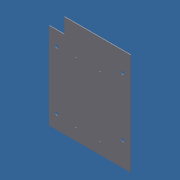
# Autodesk Inventor part: front right plate
Saved by Autodesk Inventor 2012 (Build 160160000, 160)
## iProperties
Created: 2012-03-30
Part Number: front right plate
Material: Aluminum-6061
Document SubType Name: Modeling
Designer: Edward
Density: 2.71 g/cm^3
Mass: 236.544 g
Surface Area: 1117.59 cm^2
Volume: 87.2854 cm^3
Author: Edward
Autodesk Inventor part; units mm, degrees
ref_plane "YZ Plane" through (0, 0, 0) normal (1, 0, 0) x (0, 1, 0)
ref_plane "XZ Plane" through (0, 0, 0) normal (0, 1, 0) x (-1, 0, 0)
ref_plane "XY Plane" through (0, 0, 0) normal (0, 0, 1) x (1, 0, 0)
sketch "Sketch1" plane through (0, 0, 0) normal (0, 0, 1) x (1, 0, 0)
  line L0 (0, 0) -> (213.35, 0)
  line L1 (213.35, 0) -> (213.35, 266.7)
  line L2 (213.35, 266.7) -> (0, 266.7)
  line L3 (0, 266.7) -> (0, 0)
  line L4 (0, 0) -> (41.275, 0)
  line L5 (0, 41.275) -> (0, 0)
  line L6 (0, 266.7) -> (40, 266.7)
  line L7 (40, 266.7) -> (40, 226.7)
  line L8 (40, 226.7) -> (0, 226.7)
  line L9 (0, 226.7) -> (0, 266.7)
  dimension "d0" = 266.7
  dimension "d1" = 213.35
  dimension "d4" = 40
  constraints: 20 end point, 4 parallel, 3 horizontal, 3 perpendicular
  measures "d0" distance of L2.end L0.start
  measures "d1" distance of L0.start L0.end
  measures "d4" distance of L6.end L7.end
extrude "Extrusion1" add sketch "Sketch1" along normal blind 1.5875 contours L3 L8 L7 L2 L1 L0
sketch "Sketch2" plane through (0, 0, 1.5875) normal (0, 0, 1) x (1, 0, 0)
  line L0 (213.35, 0) -> (0, 0)
  line L1 (213.35, 266.7) -> (213.35, 0)
  line L2 (40, 266.7) -> (213.35, 266.7)
  line L3 (20, 189.55) -> (20, 37.15)
  line L4 (40, 266.7) -> (40, 226.7) projected
  line L5 (40, 266.7) -> (213.35, 266.7) projected
  line L6 (0, 0) -> (0, 226.7)
  line L7 (0, 226.7) -> (40, 226.7)
  line L8 (213.35, 266.7) -> (213.35, 0) projected
  line L9 (193.35, 215.9) -> (193.35, 63.5)
  point P0 (41.275, 0)
  point P1 (126.675, 266.7)
  point P2 (20, 113.35)
  point P3 (0, 113.35)
  dimension "d9" = 152.4
  dimension "d19" = 20
  dimension "d31" = 152.4
  dimension "d32" = 20
  dimension "d33" = 50.8
  constraints: 14 end point, 3 midpoint, 2 perpendicular, 1 horizontal alignment, 1 parallel, 1 vertical alignment
  measures "d9" distance of L3.start L3.end
  measures "d19" distance between parallel lines of L6 L3
  measures "d31" distance of L9.start L9.end
  measures "d32" distance between parallel lines of L1 L9
  measures "d33" distance from line of L9.start L2
hole "Mounting Holes" at (20, 189.55, 1.5875) at (20, 37.15, 1.5875) at (193.35, 215.9, 1.5875) at (193.35, 63.5, 1.5875) direction (0, 0, -1) diameter 8.9916 end through all clearance for "Flat Head Machine Screw" size "M8" standard "Ansi Metric M Profile"
sketch "Sketch3" plane through (0, 0, 1.5875) normal (0, 0, 1) x (1, 0, 0)
  line L0 (0, 0) -> (0, 226.7) projected
  line L1 (40, 266.7) -> (213.35, 266.7) projected
  line L2 (69.85, 190.5) -> (133.35, 190.5)
  line L3 (133.35, 190.5) -> (133.35, 31.75)
  line L4 (133.35, 31.75) -> (69.85, 31.75)
  line L5 (69.85, 31.75) -> (69.85, 190.5)
  dimension "d20" = 69.85
  dimension "d21" = 63.5
  dimension "d22" = 158.75
  dimension "d23" = 76.2
  constraints: 8 end point, 2 coincident, 2 parallel, 1 horizontal, 1 perpendicular
  measures "d20" distance between parallel lines of L0 L5
  measures "d21" distance between parallel lines of L3 L5
  measures "d22" distance of L4.end L2.start
  measures "d23" distance between parallel lines of L1 L2
hole "PSU Mounting Holes" at (69.85, 190.5, 1.5875) at (133.35, 190.5, 1.5875) at (69.85, 31.75, 1.5875) at (133.35, 31.75, 1.5875) direction (0, 0, -1) diameter 4.4958 end through all clearance for "Flat Head Machine Screw (82)" size "#8" standard "Ansi Unified Screw Threads"
body "Solid1"
